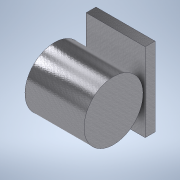
# Autodesk Inventor part: cylinder and slapper
Saved by Autodesk Inventor 2021 (Build 250183000, 183)
## iProperties
Created: 2021-03-15
Part Number: cylinder and slapper
Material: Generic
Document SubType Name: Modeling
Designer: david
Density: 1 g/cm^3
Appearance: Machined 02
Author: david
Autodesk Inventor part; units mm, degrees
ref_plane "YZ Plane" through (0, 0, 0) normal (1, 0, 0) x (0, 1, 0)
ref_plane "XZ Plane" through (0, 0, 0) normal (0, 1, 0) x (-1, 0, 0)
ref_plane "XY Plane" through (0, 0, 0) normal (0, 0, 1) x (1, 0, 0)
sketch "Sketch1" plane through (0, 0, 0) normal (1, 0, 0) x (0, 1, 0)
  circle A0 centre (63.4022, -84.5363) radius 38.1
  line L0 (114.3, -125.4125) -> (12.7, -125.4125)
  line L1 (12.7, -125.4125) -> (12.7, -138.1125)
  line L2 (12.7, -138.1125) -> (114.3, -138.1125)
  line L3 (114.3, -138.1125) -> (114.3, -125.4125)
  point P0 (0, 0)
  dimension "d0" = 76.2
  dimension "d1" = 12.7
  dimension "d2" = 101.6
  constraints: 8 end point, 2 parallel, 1 centre point, 1 horizontal, 1 perpendicular
  measures "d0" diameter of A0
  measures "d1" distance of L2.end L0.start
  measures "d2" distance of L1.end L2.end
extrude "Extrusion1" add sketch "Sketch1" along normal blind 76.2
body "Solid1"
